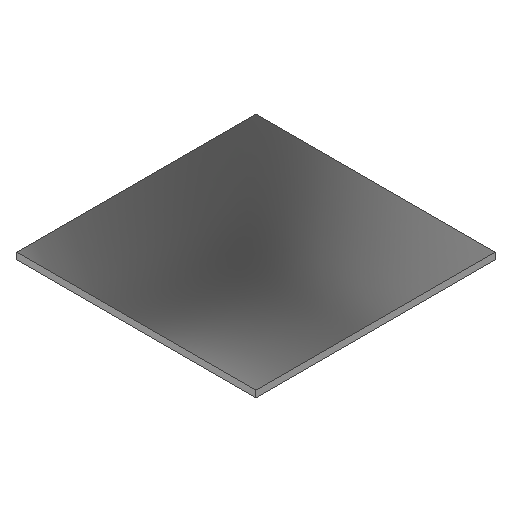
# Autodesk Inventor part: substrate_1
Saved by Autodesk Inventor 2026.2 (Build 302298000, 298)
## iProperties
Created: 2026-07-16
Part Number: substrate_1
Material: ニッケル銅合金 400
Document SubType Name: Modeling
Designer: zetsu
Density: 8.83 g/cm^3
Appearance: クロム - つや出し 黒
Author: zetsu
Autodesk Inventor part; units mm, degrees
ref_plane "YZ Plane" through (0, 0, 0) normal (1, 0, 0) x (0, 1, 0)
ref_plane "XZ Plane" through (0, 0, 0) normal (0, 1, 0) x (-1, 0, 0)
ref_plane "XY Plane" through (0, 0, 0) normal (0, 0, 1) x (1, 0, 0)
sketch "スケッチ1" plane through (0, 0, 0) normal (0, 1, 0) x (-1, 0, 0)
  line L0 (-9, 9) -> (9, 9)
  line L1 (9, 9) -> (9, -9)
  line L2 (9, -9) -> (-9, -9)
  line L3 (-9, -9) -> (-9, 9)
  line L4 (0, 0) -> (14.9737, 0) construction
  line L5 (0, 0) -> (0, -17.627) construction
  dimension "d0" = 18
  dimension "d1" = 18
  constraints: 12 end point, 2 horizontal, 2 parallel, 1 perpendicular, 1 vertical, 2 other
  measures "d0" distance of L2.end L0.start
  measures "d1" distance of L1.end L2.end
extrude "押し出し1" add sketch "スケッチ1" along normal blind 0.5
